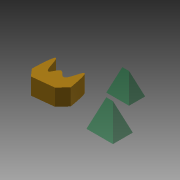
# Autodesk Inventor part: DemoSimplePart
Saved by Autodesk Inventor 2012 SP1 (Build 160190100, 190)
## iProperties
Created: 2011-09-20
Part Number: DemoSimplePart
Material: Default
Document SubType Name: Modeling
Designer: Felipe
Density: 1 g/cm^3
Author: Felipe
Autodesk Inventor part; units mm, degrees
ref_plane "YZ Plane" through (0, 0, 0) normal (1, 0, 0) x (0, 1, 0)
ref_plane "XZ Plane" through (0, 0, 0) normal (0, 1, 0) x (-1, 0, 0)
ref_plane "XY Plane" through (0, 0, 0) normal (0, 0, 1) x (1, 0, 0)
sketch "Sketch1" plane through (0, 0, 0) normal (0, 0, 1) x (1, 0, 0)
  line L0 (-42.011, 50.4132) -> (-6.6116, 50.4132)
  line L1 (-6.6116, 50.4132) -> (-6.6116, 25.4821)
  line L2 (-6.6116, 25.4821) -> (-42.011, 25.4821)
  line L3 (-42.011, 25.4821) -> (-42.011, 50.4132)
  line L4 (-8.6777, -7.8512) -> (32.5069, -7.8512)
  line L5 (32.5069, -7.8512) -> (32.5069, -38.7052)
  line L6 (32.5069, -38.7052) -> (-8.6777, -38.7052)
  line L7 (-8.6777, -38.7052) -> (-8.6777, -7.8512)
  point P0 (0, 0)
  constraints: 16 end point, 4 parallel, 2 horizontal, 2 perpendicular
extrude "Extrusion1" add sketch "Sketch1" along normal blind 50 draft -20
sketch "Sketch2" plane through (0, 0, 0) normal (0, 0, 1) x (1, 0, 0)
  spline S0 degree 4 poles (-106.3816, -25.8477) (-104.1931, 56.0594) (-90.2973, -65.9059) (-87.8849, 50.5385) (-60.7887, -55.8152) (-63.7982, 52.462) (-50.9834, -20.8633) knots 0 0 0 0 0 0.428444 0.577687 1 1 1 1 1
  line L0 (-106.3816, -25.8477) -> (-96.5552, -37.2407)
  line L1 (-96.5552, -37.2407) -> (-62.8036, -33.538)
  line L2 (-62.8036, -33.538) -> (-50.9834, -20.8633)
  point P0 (0, 0)
  point P1 (-96.5556, -4.3439)
  point P2 (-88.5804, -16.1639)
  point P3 (-81.3176, -5.7681)
  point P4 (-72.0604, -12.1762)
  point P5 (-63.943, -1.3531)
  constraints: 6 end point, 7 other
extrude "Extrusion2" add sketch "Sketch2" along normal blind 25.75 separate body
body "Solid1"
body "Solid2"
